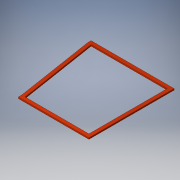
# Autodesk Inventor part: Base for Pool House
Saved by Autodesk Inventor 2016 (Build 200138000, 138)
## iProperties
Created: 2015-05-30
Part Number: Base for Pool House
Material: Wood (Oak)
Document SubType Name: Modeling
Designer: steele
Density: 0.76 g/cm^3
Appearance: White Oak - Natural Medium Gloss
Author: steele
Autodesk Inventor part; units mm, degrees
ref_plane "YZ Plane" through (0, 0, 0) normal (1, 0, 0) x (0, 1, 0)
ref_plane "XZ Plane" through (0, 0, 0) normal (0, 1, 0) x (-1, 0, 0)
ref_plane "XY Plane" through (0, 0, 0) normal (0, 0, 1) x (1, 0, 0)
sketch "Sketch1" plane through (0, 0, 0) normal (0, 1, 0) x (-1, 0, 0)
  line L0 (-44.45, 1133.475) -> (-44.45, -1133.475)
  line L1 (-44.45, -1133.475) -> (44.45, -1133.475)
  line L2 (44.45, -1133.475) -> (44.45, 1133.475)
  line L3 (44.45, 1133.475) -> (-44.45, 1133.475)
  line L4 (-44.45, 1133.475) -> (44.45, -1133.475) construction
  line L5 (-44.45, -1133.475) -> (44.45, 1133.475) construction
  line L6 (44.45, 1133.475) -> (1835.15, 1133.475)
  line L7 (1835.15, 1133.475) -> (1835.15, 1044.575)
  line L8 (1835.15, 1044.575) -> (44.45, 1044.575)
  line L9 (44.45, 1044.575) -> (44.45, 1133.475)
  line L10 (44.45, -1133.475) -> (2165.35, -1133.475)
  line L11 (2165.35, -1133.475) -> (2165.35, -1044.575)
  line L12 (2165.35, -1044.575) -> (44.45, -1044.575)
  line L13 (44.45, -1044.575) -> (44.45, -1133.475)
  point P0 (0, 0)
  dimension "d0" = 88.9
  dimension "d1" = 2266.95
  dimension "d2" = 88.9
  dimension "d3" = 1879.6
  dimension "d4" = 88.9
  dimension "d5" = 2209.8
  constraints: 28 end point, 6 parallel, 3 perpendicular, 2 horizontal, 2 midpoint, 1 vertical
  measures "d0" distance of L1.end L0.end
  measures "d1" distance of L0.start L0.end
  measures "d2" distance of L6.end L7.end
  measures "d3" distance between parallel lines of L7 L0
  measures "d4" distance between parallel lines of L12 L10
  measures "d5" distance between parallel lines of L11 L0
extrude "Extrusion1" add sketch "Sketch1" along normal blind 38.1
sketch "Sketch2" plane through (0, 38.1, 0) normal (0, 1, 0) x (1, 0, 0)
  line L0 (-44.45, -1044.575) -> (-1835.15, -1044.575) projected
  line L1 (-2165.35, 1044.575) -> (-1835.15, -1044.575)
  line L2 (-1835.15, -1044.575) -> (-1745.1464, -1044.575)
  line L3 (-1745.1464, -1044.575) -> (-2075.3464, 1044.575)
  line L4 (-2165.35, 1044.575) -> (-44.45, 1044.575) projected
  line L5 (-2075.3464, 1044.575) -> (-2165.35, 1044.575)
  point P0 (0, 0)
  dimension "d8" = 88.9
  dimension "d9" = 98.982
  dimension "d10" = 81.018
  constraints: 8 end point, 1 collinear, 1 parallel, 1 point on line
  measures "d8" distance between parallel lines of L3 L1
  measures "d9" angle of L0 L1
  measures "d10" angle of L1 L4
extrude "Extrusion2" add sketch "Sketch2" against normal blind 38.1
body "Solid1"
